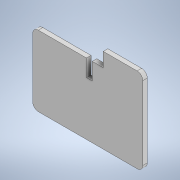
# Autodesk Inventor part: pcb_balun_bottom
Saved by Autodesk Inventor 2020.2 (Build 242310000, 310)
## iProperties
Created: 2020-09-26
Part Number: pcb_balun_bottom
Material: Generic
Document SubType Name: Modeling
Designer: Krishna Makhija
Density: 1 g/cm^3
Appearance: Default
Author: Krishna Makhija
Autodesk Inventor part; units mm, degrees
ref_plane "YZ Plane" through (0, 0, 0) normal (1, 0, 0) x (0, 1, 0)
ref_plane "XZ Plane" through (0, 0, 0) normal (0, 1, 0) x (-1, 0, 0)
ref_plane "XY Plane" through (0, 0, 0) normal (0, 0, 1) x (1, 0, 0)
sketch "Sketch5" plane through (0, 0, 0) normal (0, 0, 1) x (1, 0, 0)
  line L0 (19.5001, -12.4998) -> (-19.5001, -12.4998)
  line L1 (-19.5001, -12.4998) -> (-19.5001, 12.4998)
  line L2 (19.5001, 12.4998) -> (19.5001, -12.4998)
  line L3 (19.5001, -12.4998) -> (-19.5001, 12.4998) construction
  line L4 (-19.5001, -12.4998) -> (19.5001, 12.4998) construction
  line L5 (5.5001, 12.4998) -> (5.5001, 17.4994)
  line L6 (5.5001, 17.4994) -> (19.5001, 17.4994)
  line L7 (19.5001, 17.4994) -> (19.5001, 12.4998)
  line L8 (1.6001, 6.4997) -> (-0.4001, 6.4997)
  line L9 (-0.4001, 6.4997) -> (-0.4001, 12.4998)
  line L10 (1.6001, 12.4998) -> (1.6001, 6.4997)
  line L11 (1.6001, 6.4997) -> (-0.4001, 12.4998) construction
  line L12 (-0.4001, 6.4997) -> (1.6001, 12.4998) construction
  line L13 (-19.5001, 12.4998) -> (-0.4001, 12.4998)
  line L14 (1.6001, 12.4998) -> (5.5001, 12.4998)
  constraints: 30 end point, 3 horizontal, 3 parallel, 2 perpendicular, 1 collinear
extrude "Extrusion4" add sketch "Sketch5" along normal blind 1.6
fillet "Fillet4" radius 2 4 edges at (19.5001, 17.4994, 0.8) (19.5001, -12.4998, 0.8) (-19.5001, -12.4998, 0.8) (-19.5001, 12.4998, 0.8)
body "Solid4"
